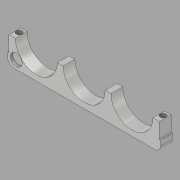
# Autodesk Inventor part: Tube Holder Halve 3
Saved by Autodesk Inventor 2017 (Build 210142000, 142)
## iProperties
Created: 2016-12-06
Part Number: Tube Holder Halve 3
Material: Aluminum 6061-AHC
Document SubType Name: Modeling
Designer: qupec
Density: 2.7 g/cm^3
Appearance: Aluminum - Dark
Mass: 40.9656 g
Surface Area: 72.5902 cm^2
Volume: 15.1725 cm^3
Author: qupec
Autodesk Inventor part; units mm, degrees
ref_plane "YZ Plane" through (0, 0, 0) normal (1, 0, 0) x (0, 1, 0)
ref_plane "XZ Plane" through (0, 0, 0) normal (0, 1, 0) x (-1, 0, 0)
ref_plane "XY Plane" through (0, 0, 0) normal (0, 0, 1) x (1, 0, 0)
sketch "Sketch1" plane through (0, 0, 0) normal (0, 0, 1) x (1, 0, 0)
  line L0 (-41.148, 14.2875) -> (41.148, 14.2875)
  line L1 (41.148, 14.2875) -> (41.148, -14.2875)
  line L2 (41.148, -14.2875) -> (-41.148, -14.2875)
  line L3 (-41.148, -14.2875) -> (-41.148, 14.2875)
  point P0 (0, 0)
  dimension "d0" = 82.296
  dimension "d1" = 41.148
  dimension "d2" = 14.2875
  dimension "d3" = 28.575
  constraints: 8 end point, 2 parallel, 1 horizontal, 1 perpendicular
  measures "d0" distance of L0.start L0.end
  measures "d1" distance from line of point (0, 0) L3
  measures "d2" distance from line of point (0, 0) L2
  measures "d3" distance of L2.end L0.start
extrude "Extrusion1" add sketch "Sketch1" along normal mid plane 6.35
sketch "Sketch2" plane through (0, 0, 3.175) normal (0, 0, 1) x (1, 0, 0)
  circle A0 centre (-25.781, 0) radius 11.303
  circle A1 centre (0, 0) radius 11.303
  line L0 (41.148, -14.2875) -> (41.148, 14.2875) projected
  circle A2 centre (25.781, 0) radius 11.303
  line L1 (-41.148, 14.2875) -> (-41.148, -14.2875) projected
  line L2 (-41.148, 0) -> (41.148, 0) construction
  line L3 (41.148, 14.2875) -> (-41.148, 14.2875) projected
  point P0 (0, 0)
  dimension "d6" = 22.606
  dimension "d9" = 22.606
  dimension "d11" = 22.606
  dimension "d14" = 25.781
  dimension "d21" = 82.296
  dimension "d22" = 25.781
  dimension "d50" = 0
  dimension "d97" = 3.175
  constraints: 3 centre point, 3 midpoint, 2 end point, 1 point on line
  measures "d6" diameter of A0
  measures "d9" diameter of A1
  measures "d11" diameter of A2
  measures "d14" distance of A1.centre A0.centre
  measures "d21" distance of L0.end L1.start
  measures "d22" distance of A2.centre A1.centre
  measures "d50" distance of point (0, 0) A1.centre
sketch "Sketch4" plane through (-41.148, -14.2875, -3.175) normal (-1, 0, 0) x (0, 0, 1)
  line L0 (0, 0) -> (0, 28.575) projected
  line L1 (6.35, 28.575) -> (6.35, 0) projected
  line L2 (0, 22.6695) -> (6.35, 22.6695)
  line L3 (6.35, 22.6695) -> (6.35, 5.9055)
  line L4 (6.35, 5.9055) -> (0, 5.9055)
  line L5 (0, 5.9055) -> (0, 22.6695)
  point P0 (3.175, 14.2875)
  dimension "d30" = 8.382
  dimension "d31" = 16.764
  constraints: 8 end point, 2 parallel, 1 horizontal, 1 perpendicular, 1 point on line, 2 other
  measures "d30" distance from line of point (3.175, 14.288) L4
  measures "d31" distance between parallel lines of L4 L2
extrude "Extrusion3" cut sketch "Sketch4" against normal blind 0.635
mirror "Mirror1" about plane through (0, 0, 0) normal (1, 0, 0) of "Extrusion3"
sketch "Sketch5" plane through (0, 0, 3.175) normal (0, 0, 1) x (1, 0, 0)
  circle A0 centre (0, 9.7155) radius 3.175 construction
  line L0 (41.148, 14.2875) -> (-41.148, 14.2875) projected
  line L1 (-18.3944, 20.454) -> (40.513, 0) construction
  line L2 (40.513, 8.382) -> (40.513, -8.382) projected
  circle A1 centre (2.6968, 17.4822) radius 3.175 construction
  circle A2 centre (35.941, 1.5875) radius 3.175 construction
  circle A3 centre (-35.941, 26.5465) radius 3.175 construction
  line L3 (-40.513, 8.382) -> (-40.513, -8.382) projected
  circle A4 centre (36.576, 9.7155) radius 3.175
  circle A5 centre (-36.576, -9.7155) radius 3.175
  line L4 (41.148, 8.382) -> (41.148, 14.2875) projected
  line L5 (-41.148, -14.2875) -> (41.148, -14.2875) projected
  line L6 (-41.148, -14.2875) -> (-41.148, -8.382) projected
  point P0 (0, 0)
  dimension "d34" = 6.35
  dimension "d35" = 4.572
  dimension "d53" = 6.35
  dimension "d54" = 6.35
  dimension "d55" = 4.572
  dimension "d56" = 4.572
  dimension "d57" = 12.7
  dimension "d58" = 6.35
  dimension "d59" = 6.35
  dimension "d60" = 4.572
  dimension "d61" = 4.572
  dimension "d62" = 4.572
  dimension "d63" = 4.572
  constraints: 6 centre point, 2 end point, 2 point on line, 1 midpoint, 1 symmetric about line, 1 other
  measures "d34" diameter of A0
  measures "d35" distance from line of L0 A0.centre
  measures "d53" diameter of A2
  measures "d54" diameter of A3
  measures "d55" distance from line of L2 A2.centre
  measures "d56" distance from line of L3 A3.centre
  measures "d57" distance from line of L0 A2.centre
  measures "d58" diameter of A4
  measures "d59" diameter of A5
  measures "d60" distance from line of L4 A4.centre
  measures "d61" distance from line of L0 A4.centre
  measures "d62" distance from line of L5 A5.centre
  measures "d63" distance from line of L6 A5.centre
extrude "Extrusion4" cut sketch "Sketch5" against normal blind 1.27
sketch "Sketch7" plane through (-41.148, -14.2875, 3.175) normal (0, -1, 0) x (1, 0, 0)
  line L0 (27.178, -14.605) -> (55.118, -14.605)
  line L1 (55.118, -14.605) -> (55.118, 8.255)
  line L2 (55.118, 8.255) -> (27.178, 8.255)
  line L3 (27.178, 8.255) -> (27.178, -14.605)
  point P0 (41.148, -3.175)
  dimension "d39" = 27.94
  dimension "d40" = 22.86
  dimension "d41" = 11.43
  dimension "d42" = 13.97
  constraints: 8 end point, 2 parallel, 1 horizontal, 1 perpendicular
  measures "d39" distance of L0.start L0.end
  measures "d40" distance of L2.end L0.start
  measures "d41" distance from line of point (41.148, -3.175) L0
  measures "d42" distance from line of point (41.148, -3.175) L1
extrude "Extrusion5" [suppressed]
sketch "Sketch8" plane through (0, 0, -3.175) normal (0, 0, -1) x (-1, 0, 0)
  line L0 (-41.148, 14.2875) -> (41.148, 14.2875) projected
  line L1 (15.6718, 14.2875) -> (-15.6718, 14.2875)
  line L2 (-15.6718, 14.2875) -> (-15.6718, 52.3875)
  line L3 (-15.6718, 52.3875) -> (15.6718, 52.3875)
  line L4 (15.6718, 52.3875) -> (15.6718, 14.2875)
  point P0 (0, 0)
  dimension "d45" = 31.3436
  dimension "d46" = 38.1
  dimension "d47" = 15.6718
  constraints: 8 end point, 2 parallel, 1 horizontal, 1 perpendicular, 1 point on line
  measures "d45" distance between parallel lines of L2 L4
  measures "d46" distance between parallel lines of L0 L3
  measures "d47" distance from line of point (0, 0) L4
extrude "Extrusion6" add sketch "Sketch8" against normal up to surface (6.35 mm away)
extrude "Extrusion7" cut sketch "Sketch2" against normal blind 25.4
sketch "Sketch9" plane through (-15.6718, 52.3875, -3.175) normal (0, 1, 0) x (1, 0, 0)
  line L0 (-25.4762, -6.35) -> (56.8198, -6.35) projected
  line L1 (3.1718, -6.35) -> (28.1718, -6.35)
  line L2 (28.1718, -6.35) -> (28.1718, -3.175)
  line L3 (28.1718, -3.175) -> (3.1718, -3.175)
  line L4 (3.1718, -3.175) -> (3.1718, -6.35)
  point P0 (15.6718, -3.175)
  dimension "d64" = 3.175
  dimension "d65" = 25
  dimension "d66" = 12.5
  constraints: 8 end point, 2 parallel, 1 horizontal, 1 perpendicular, 1 point on line
  measures "d64" distance of L3.end L1.start
  measures "d65" distance of L2.end L3.end
  measures "d66" distance from line of point (15.672, -3.175) L4
extrude "Extrusion8" cut sketch "Sketch9" against normal blind 0.9
sketch "Sketch13" plane through (0, 0, 3.175) normal (0, 0, 1) x (1, 0, 0)
  line L0 (-15.6718, 52.3875) -> (-12.5, 52.3875) projected
  line L1 (-12.5, 52.3875) -> (12.5, 52.3875) projected
  line L2 (12.5, 52.3875) -> (15.6718, 52.3875) projected
  line L3 (15.6718, 52.3875) -> (15.6718, 14.2875) projected
  line L4 (-15.6718, 14.2875) -> (-15.6718, 52.3875) projected
  line L5 (-15.6718, 14.2875) -> (-41.148, 14.2875) projected
  line L6 (41.148, 14.2875) -> (15.6718, 14.2875) projected
  line L7 (41.148, 8.382) -> (41.148, 14.2875) projected
  line L8 (-41.148, 14.2875) -> (-41.148, 8.382) projected
  line L9 (-41.148, 8.382) -> (-40.513, 8.382) projected
  line L10 (40.513, 8.382) -> (41.148, 8.382) projected
  line L11 (-40.513, 8.382) -> (-40.513, 0)
  line L12 (-40.513, 8.382) -> (-40.513, -8.382) projected
  line L13 (-40.513, 0) -> (40.513, 0)
  line L14 (40.513, 8.382) -> (40.513, -8.382) projected
  line L15 (40.513, 0) -> (40.513, 8.382)
  point P0 (0, 0)
  constraints: 6 end point, 1 collinear, 1 horizontal, 1 midpoint
extrude "Extrusion11" cut sketch "Sketch13" against normal through all
sketch "Sketch14" plane through (-40.513, 0, 3.175) normal (0, 1, 0) x (1, 0, 0)
  line L0 (7.112, 0) -> (0.762, 0) projected
  line L1 (7.112, 1.27) -> (0.762, 1.27) projected
  line L2 (3.429, 6.35) -> (3.429, 0) projected
  line L3 (0, 6.35) -> (3.429, 6.35) projected
  line L4 (0, 0) -> (0, 6.35) projected
  line L5 (3.429, 0) -> (0, 0) projected
  circle A0 centre (1.7145, 3.81) radius 1.5494
  point P0 (40.513, 3.175)
  dimension "d84" = 3.0988
  dimension "d85" = 3.429
  dimension "d86" = 5.08
  dimension "d87" = 2.54
  dimension "d88" = 1.7145
  constraints: 1 centre point
  measures "d84" diameter of A0
  measures "d85" distance of L3.start L2.start
  measures "d86" distance between parallel lines of L3 L1
  measures "d87" distance from line of L3 A0.centre
  measures "d88" distance from line of L2 A0.centre
extrude "Extrusion12" cut sketch "Sketch14" against normal blind 11.43 contours A0
mirror "Mirror3" about plane through (0, 0, 0) normal (1, 0, 0) of "Extrusion12"
thread "Thread3" size "5-40 UNC" class "2B" standard "ANSI Unified Screw Threads" full length
thread "Thread4" size "5-40 UNC" class "2B" standard "ANSI Unified Screw Threads" full length
fillet "Fillet1" radius 3.175 2 edges at (41.148, -14.2875, 0) (-41.148, -14.2875, 0)
equation "\"d1\" = 0.5 * d0"
equation "\"d2\" = 0.5 * d3"
equation "\"d9\" = d7"
equation "\"d11\" = d9"
equation "\"d22\" = d14"
equation "\"d30\" = 0.5 * d31"
equation "\"d41\" = 0.5 * d40"
equation "\"d42\" = 0.5 * d39"
equation "\"d47\" = 0.5 * d45"
equation "\"d66\" = 0.5 * d65"
equation "\"d87\" = 0.5 * d86"
equation "\"d88\" = 0.5 * d85"
equation "\"d7\" = d6"
body "Solid1"
